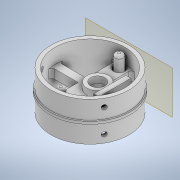
# Autodesk Inventor part: Verbindungsring_2_2
Saved by Autodesk Inventor 2020 (Build 240168000, 168)
## iProperties
Created: 2022-02-05
Part Number: Verbindungsring_2_2
Material: Generisch
Document SubType Name: Modeling
Designer: sp
Density: 1 g/cm^3
Appearance: Vorgabe
Author: sp
## iProperties of the stored document _3D-Druck.ipt
Created: 2022-05-01
Part Number: _3D-Druck
Material: Generisch
Document SubType Name: Modeling
Designer: sp
Density: 1 g/cm^3
Appearance: Vorgabe
Author: sp
Autodesk Inventor part; units mm, degrees
ref_plane "YZ Plane" through (0, 0, 0) normal (1, 0, 0) x (0, 1, 0)
ref_plane "XZ Plane" through (0, 0, 0) normal (0, 1, 0) x (-1, 0, 0)
sketch "Skizze5" plane through (0, 0, 0) normal (0, 1, 0) x (-1, 0, 0)
  circle A0 centre (0, 0) radius 27
  circle A1 centre (0, 0) radius 31
  dimension "d23" = 62
  dimension "d24" = 54
  constraints: 2 centre point, 2 coincident
  measures "d23" diameter of A1
  measures "d24" diameter of A0
extrude "Extrusion4" add sketch "Skizze5" along normal mid plane 2
sketch "Skizze6" plane through (0, 0, 0) normal (0, 1, 0) x (-1, 0, 0)
  circle A0 centre (0, 0) radius 27
  circle A1 centre (0, 0) radius 30
  dimension "d27" = 54
  dimension "d28" = 60
  constraints: 2 centre point, 2 coincident
  measures "d27" diameter of A0
  measures "d28" diameter of A1
extrude "Extrusion5" add sketch "Skizze6" along normal mid plane 30
ref_plane "Arbeitsebene5" through (0, 0, -30) normal (0, 0, 1) x (1, 0, 0)
sketch "Skizze7" plane through (0, 0, -30) normal (0, 0, 1) x (1, 0, 0)
  circle A0 centre (0, -9) radius 1.75
  circle A1 centre (0, 9) radius 1.75
  line L0 (-34.5015, 0) -> (40.4508, 0) construction
  point P0 (0, 0)
  dimension "d32" = 3.5
  dimension "d33" = 3.5
  dimension "d34" = 18
  constraints: 2 centre point, 2 end point, 1 horizontal, 1 point on line, 1 symmetric about line
  measures "d32" diameter of A0
  measures "d33" diameter of A1
  measures "d34" distance of A1.centre A0.centre
extrude "Extrusion6" cut sketch "Skizze7" along normal blind 5
pattern_circular "Runde Anordnung2" count 3 over 360 about axis through (0, -10, 0) along (0, 1, 0) of "Extrusion6"
sketch "Skizze8" plane through (0, 0, 0) normal (0, 1, 0) x (-1, 0, 0)
  line L0 (-16.7844, 0) -> (18.1163, 0) construction
  line L1 (0, -12.3348) -> (0, 12.3348) construction
  circle A0 centre (0, -22.5) radius 1.75
  circle A1 centre (0, 22.5) radius 1.75
  circle A2 centre (0, -22.5) radius 5
  circle A3 centre (0, 22.5) radius 5
  line L2 (-5, -22.5) -> (5, -22.5)
  line L3 (5, -22.5) -> (5, 22.5)
  line L4 (5, 22.5) -> (-5, 22.5)
  line L5 (-5, 22.5) -> (-5, -22.5)
  circle A4 centre (0, 0) radius 27.0734
  line L6 (-29, -3) -> (29, -3)
  line L7 (29, -3) -> (29, 3)
  line L8 (29, 3) -> (-29, 3)
  line L9 (-29, 3) -> (-29, -3)
  line L10 (6, -27.5) -> (-6, -27.5)
  line L11 (-6, -27.5) -> (-6, 27.5)
  line L12 (-6, 27.5) -> (6, 27.5)
  line L13 (6, 27.5) -> (6, -27.5)
  point P0 (5, -3)
  point P1 (26.9066, -3)
  point P2 (26.9066, 3)
  point P3 (5, 3)
  point P4 (2.215, 26.9826)
  point P5 (-2.215, 26.9826)
  point P6 (-5, 3)
  point P7 (-26.9066, 3)
  point P8 (-26.9066, -3)
  point P9 (-5, -3)
  point P10 (-2.215, -26.9826)
  point P11 (2.215, -26.9826)
  point P12 (-6, 3)
  point P13 (6, 3)
  point P14 (6, -3)
  point P15 (-6, -3)
  dimension "d43" = 10
  dimension "d44" = 10
  dimension "d40" = 3.5
  dimension "d41" = 3.5
  dimension "d42" = 45
  dimension "d45" = 6
  dimension "d46" = 58
  dimension "d59" = 10
  dimension "d60" = 12
  constraints: 28 end point, 6 parallel, 4 horizontal, 3 centre point, 3 coincident, 3 perpendicular, 3 point on line, 1 midpoint, 1 symmetric about line, 1 vertical, 9 other
  measures "d40" diameter of A0
  measures "d41" diameter of A1
  measures "d42" distance of A1.centre A0.centre
  measures "d45" distance of L6.end L7.end
  measures "d46" distance of L7.end L8.end
  measures "d59" distance between parallel lines of L3 L5
  measures "d60" distance between parallel lines of L13 L11
extrude "Extrusion7" add sketch "Skizze8" along normal mid plane 7 contours L2 A0 | L2 A2 A4 A0 | A0 L2 A2 | A0 L2 | L3 L6 L13 A4 A2 | A2 L5 L6 L3 | A2 A4 L11 L6 L5 | A4 L13 L10 A2 | A2 A4 | L6 L5 L8 L3 | L3 L8 L13 L6 | A2 L10 L11 A4 | L6 L11 L8 L5 | L8 L5 A3 L3 | L3 A3 A4 L13 L8 | L13 L8 A4 L6 | L8 L11 A4 A3 L5 | L6 A4 L8 L11 | L4 A1 A3 A4 | A3 L4 A1 | A4 A3 | A3 L12 L13 A4 | L4 A1 | A1 L4 | A4 L11 L12 A3
fillet "Rundung3" radius 2 16 edges at (26.8328, 2.25, -3) (26.8328, -2.25, -3) (26.8328, -0.5, -3) (26.8328, 0.5, -3) (26.8328, 2.25, 3) (26.8328, -2.25, 3) (26.8328, 0.5, 3) (26.8328, -0.5, 3) (-26.8328, 2.25, -3) (-26.8328, -2.25, -3) (-26.8328, 0.5, -3) (-26.8328, -0.5, -3) (-26.8328, 2.25, 3) (-26.8328, -2.25, 3) (-26.8328, -0.5, 3) (-26.8328, 0.5, 3)
sketch "Skizze9" plane through (0, 3.5, 0) normal (0, 1, 0) x (1, 0, 0)
  circle A0 centre (0, -22.5) radius 1.75 projected
  circle A1 centre (0, -22.5) radius 3
  circle A2 centre (0, 22.5) radius 1.75 projected
  circle A3 centre (0, 22.5) radius 3
  point P0 (0, 0)
  dimension "d52" = 6
  dimension "d53" = 6
  constraints: 2 centre point, 2 coincident
  measures "d52" diameter of A3
  measures "d53" diameter of A1
extrude "Extrusion8" add sketch "Skizze9" along normal blind 10 contours A0 | A1 | A2 | A3
fillet "Rundung5" radius 2 2 edges at (-3, 13.5, -22.5) (-3, 13.5, 22.5)
fillet "Rundung6" radius 2 4 edges at (6, 0, -26.3249) (-6, 0, -26.3249) (6, 0, 26.3249) (-6, 0, 26.3249)
sketch "Skizze11" plane through (0, 3.5, 0) normal (0, 1, 0) x (1, 0, 0)
  circle A0 centre (0, 22.5) radius 1 projected
  circle A1 centre (0, 22.5) radius 3
  circle A2 centre (0, 22.5) radius 4.1
  circle A3 centre (0, -22.5) radius 1 projected
  circle A4 centre (0, -22.5) radius 3
  circle A5 centre (0, -22.5) radius 4.1
  point P0 (0, 0)
  dimension "d62" = 8.2
  dimension "d63" = 6
  dimension "d64" = 8.2
  constraints: 4 centre point, 4 coincident
  measures "d62" diameter of A2
  measures "d63" diameter of A4
  measures "d64" diameter of A5
extrude "Extrusion10" cut sketch "Skizze11" against normal blind 3 contours A2 | A5
fillet "Rundung7" radius 0.5 2 edges at (-4.1, 3.5, -22.5) (-4.1, 3.5, 22.5)
sketch "Skizze12" plane through (0, 3.5, 0) normal (0, 1, 0) x (1, 0, 0)
  line L0 (15, -12.3187) -> (19, -12.3187)
  line L1 (19, -12.3187) -> (19, 12.6813)
  line L2 (19, 12.6813) -> (15, 12.6813)
  line L3 (15, 12.6813) -> (15, -12.3187)
  line L4 (-53.0839, 0.1813) -> (74.1241, 0.1813) construction
  line L5 (0, -55.5359) -> (0, 55.8985) construction
  point P0 (0, 0)
  point P1 (0, 0.1813)
  dimension "d68" = 25
  dimension "d69" = 4
  dimension "d70" = 15
  constraints: 12 end point, 2 horizontal, 2 parallel, 2 point on line, 1 midpoint, 1 perpendicular, 1 vertical, 1 other
  measures "d68" distance of L2.end L0.start
  measures "d69" distance of L1.end L2.end
  measures "d70" distance between parallel lines of L5 L3
extrude "Extrusion11" add sketch "Skizze12" along normal mid plane 15
sketch "Skizze13" plane through (0, 3.5, 0) normal (0, 1, 0) x (1, 0, 0)
  circle A0 centre (6, 0) radius 5.5
  circle A1 centre (6, 0) radius 8.3127
  point P0 (0, 0)
  dimension "d73" = 11
  dimension "d74" = 6
  constraints: 2 centre point, 1 coincident
  measures "d73" diameter of A0
  measures "d74" distance of point (0, 0) A0.centre
extrude "Extrusion12" add sketch "Skizze13" along normal blind 5
